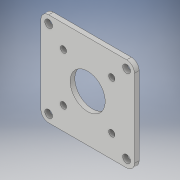
# Autodesk Inventor part: TurntableMotorBracket
Saved by Autodesk Inventor 2019.3 (Build 233278000, 278)
## iProperties
Created: 2019-07-07
Part Number: TurntableMotorBracket
Material: Generic
Document SubType Name: Modeling
Designer: mark
Density: 1 g/cm^3
Appearance: Default
Author: mark
Autodesk Inventor part; units mm, degrees
ref_plane "YZ Plane" through (0, 0, 0) normal (1, 0, 0) x (0, 1, 0)
ref_plane "XZ Plane" through (0, 0, 0) normal (0, 1, 0) x (-1, 0, 0)
ref_plane "XY Plane" through (0, 0, 0) normal (0, 0, 1) x (1, 0, 0)
sketch "Sketch1" plane through (0, 0, 0) normal (0, 0, 1) x (1, 0, 0)
  line L0 (-30, 30) -> (30, 30)
  line L1 (30, 30) -> (30, -30)
  line L2 (30, -30) -> (-30, -30)
  line L3 (-30, -30) -> (-30, 30)
  circle A0 centre (-15.5, 15.5) radius 2
  circle A1 centre (-15.5, -15.5) radius 2
  circle A2 centre (15.5, -15.5) radius 2
  circle A3 centre (15.5, 15.5) radius 2
  circle A4 centre (0, 0) radius 11.25
  circle A5 centre (-25, 25) radius 2.5
  circle A6 centre (25, 25) radius 2.5
  circle A7 centre (-25, -25) radius 2.5
  circle A8 centre (25, -25) radius 2.5
  dimension "d0" = 4
  dimension "d1" = 4
  dimension "d2" = 4
  dimension "d3" = 4
  dimension "d4" = 22.5
  dimension "d5" = 31
  dimension "d6" = 31
  dimension "d7" = 31
  dimension "d8" = 31
  dimension "d9" = 15.5
  dimension "d10" = 15.5
  dimension "d11" = 15.5
  dimension "d12" = 15.5
  dimension "d13" = 60
  dimension "d14" = 60
  dimension "d15" = 30
  dimension "d16" = 30
  dimension "d17" = 5
  dimension "d18" = 5
  dimension "d19" = 5
  dimension "d20" = 5
  dimension "d21" = 50
  dimension "d22" = 50
  dimension "d23" = 50
  dimension "d24" = 50
  dimension "d25" = 5
  dimension "d26" = 5
  dimension "d27" = 5
  dimension "d28" = 5
  constraints: 9 centre point, 8 end point, 2 horizontal, 2 vertical, 1 coincident
  measures "d0" diameter of A0
  measures "d1" diameter of A1
  measures "d2" diameter of A2
  measures "d3" diameter of A3
  measures "d4" diameter of A4
  measures "d5" distance of A3.centre A0.centre
  measures "d6" distance of A1.centre A0.centre
  measures "d7" distance of A1.centre A2.centre
  measures "d8" distance of A2.centre A3.centre
  measures "d9" horizontal distance of A3.centre point (0, 0)
  measures "d10" horizontal distance of point (0, 0) A3.centre
  measures "d11" horizontal distance of point (0, 0) A1.centre
  measures "d12" horizontal distance of A1.centre point (0, 0)
  measures "d13" distance between parallel lines of L1 L3
  measures "d14" distance between parallel lines of L2 L0
  measures "d15" distance from line of L2 point (0, 0)
  measures "d16" distance from line of L3 point (0, 0)
  measures "d17" diameter of A5
  measures "d18" diameter of A6
  measures "d19" diameter of A7
  measures "d20" diameter of A8
  measures "d21" distance of A6.centre A5.centre
  measures "d22" distance of A7.centre A5.centre
  measures "d23" distance of A8.centre A7.centre
  measures "d24" distance of A8.centre A6.centre
  measures "d25" distance from line of L1 A6.centre
  measures "d26" distance from line of L0 A6.centre
  measures "d27" distance from line of L2 A7.centre
  measures "d28" distance from line of L3 A7.centre
extrude "Extrusion1" add sketch "Sketch1" along normal blind 3
fillet "Fillet1" radius 5 4 edges at (30, 30, 1.5) (30, -30, 1.5) (-30, 30, 1.5) (-30, -30, 1.5)
body "Solid1"
